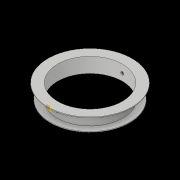
# Autodesk Inventor part: Layer2_Ref
Saved by Autodesk Inventor 2017 (Build 210142000, 142)
## iProperties
Created: 2017-01-16
Part Number: Layer2_Ref
Material: Generic
Document SubType Name: Modeling
Designer: David Kopala
Density: 1 g/cm^3
Appearance: Default
Author: David Kopala
Autodesk Inventor part; units mm, degrees
ref_plane "YZ Plane" through (0, 0, 0) normal (1, 0, 0) x (0, 1, 0)
ref_plane "XZ Plane" through (0, 0, 0) normal (0, 1, 0) x (-1, 0, 0)
ref_plane "XY Plane" through (0, 0, 0) normal (0, 0, 1) x (1, 0, 0)
sketch "Sketch1" plane through (0, 0, 0) normal (1, 0, 0) x (0, 1, 0)
  line L0 (0, 0) -> (50.8, 0)
  line L1 (0, 138.1125) -> (26.719, 138.1125)
  line L2 (0, 138.1125) -> (0, 169.8625)
  line L3 (0, 169.8625) -> (3.175, 169.8625)
  line L4 (3.175, 169.8625) -> (3.175, 141.2875)
  line L5 (3.175, 141.2875) -> (60.325, 141.2875)
  line L6 (60.325, 141.2875) -> (60.325, 179.3875)
  line L7 (60.325, 179.3875) -> (63.5, 179.3875)
  line L8 (63.5, 179.3875) -> (63.5, 138.1125)
  line L9 (63.5, 138.1125) -> (26.719, 138.1125)
  point P0 (62.1333, 179.3875)
  dimension "d0" = 50.8
  dimension "d1" = 138.1125
  dimension "d2" = 31.75
  dimension "d3" = 3.175
  dimension "d4" = 3.175
  dimension "d5" = 57.15
  dimension "d6" = 38.1
  dimension "d7" = 3.175
  constraints: 20 end point, 4 perpendicular, 3 horizontal, 1 collinear, 1 parallel, 1 point on line, 1 vertical
  measures "d0" distance of L0.start L0.end
  measures "d1" distance between parallel lines of L0 L1
  measures "d2" distance of L1.start L2.end
  measures "d3" distance of L2.end L3.end
  measures "d4" distance from line of L1 L4.end
  measures "d5" distance of L4.end L5.end
  measures "d6" distance of L5.end L6.end
  measures "d7" distance of L6.end L7.end
revolve "Revolution1" add sketch "Sketch1" angle 360 about axis through (0, 0, 0) along (0, 1, 0)
ref_plane "Work Plane1" through (0, 62.1333, 179.3875) normal (0, 0, 1) x (1, 0, 0)
sketch "Sketch2" plane through (0, 62.1333, 179.3875) normal (0, 0, 1) x (1, 0, 0)
  circle A0 centre (0, -32.8344) radius 6.35
  line L0 (169.8625, -58.9583) -> (-169.8625, -58.9583) projected
  point P0 (0, -62.1333)
  dimension "d9" = 12.7
  dimension "d10" = 26.1239
  constraints: 1 centre point
  measures "d9" diameter of A0
  measures "d10" distance from line of A0.centre L0
extrude "Extrusion1" cut sketch "Sketch2" against normal through all
body "Solid1"
